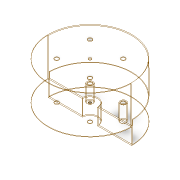
# Autodesk Inventor part: WaterproofCover
Saved by Autodesk Inventor 2018 (Build 220112000, 112)
## iProperties
Created: 2017-12-09
Part Number: WaterproofCover
Material: Polyethylene, Low Density
Document SubType Name: Modeling
Designer: Udara Wanasinghe
Mass: 493.701 g
Surface Area: 5556.42 cm^2
Volume: 552.239 cm^3
Density: 0.894 g/cm^3
Appearance: Smooth - Off-White
Author: Udara Wanasinghe
Autodesk Inventor part; units mm, degrees
ref_plane "YZ Plane" through (0, 0, 0) normal (1, 0, 0) x (0, 1, 0)
ref_plane "XZ Plane" through (0, 0, 0) normal (0, 1, 0) x (-1, 0, 0)
ref_plane "XY Plane" through (0, 0, 0) normal (0, 0, 1) x (1, 0, 0)
sketch "Sketch1" plane through (0, 0, 0) normal (0, 1, 0) x (-1, 0, 0)
  circle A0 centre (0, 0) radius 156
  dimension "d1" = 312
  constraints: 1 centre point
  measures "d1" diameter of A0
extrude "Extrusion1" add sketch "Sketch1" along normal blind 144
ref_plane "Work Plane1" through (0, 2, 0) normal (0, -1, 0) x (1, 0, 0)
sketch "Sketch2" plane through (0, 2, 0) normal (0, -1, 0) x (1, 0, 0)
  circle A0 centre (0, 0) radius 154
  dimension "d5" = 308
  constraints: 1 centre point, 1 coincident
  measures "d5" diameter of A0
extrude "Extrusion2" cut sketch "Sketch2" against normal blind 140
sketch "Sketch3" plane through (0, 144, 0) normal (0, 1, 0) x (1, 0, 0)
  circle A0 centre (0, 0) radius 5
  dimension "d8" = 10
  constraints: 1 centre point, 1 coincident
  measures "d8" diameter of A0
extrude "Extrusion3" cut sketch "Sketch3" against normal through all
sketch "Sketch5" plane through (0, 144, 0) normal (0, 1, 0) x (1, 0, 0)
  line L0 (0, 156) -> (0, -156) construction
  line L1 (156, 0) -> (-156, 0) construction
  circle A0 centre (62.132, -62.132) radius 7.5
  line L2 (62.132, -62.132) -> (0, -62.132) construction
  line L3 (62.132, -62.132) -> (62.132, 0) construction
  line L4 (62.132, -62.132) -> (106.066, -106.066) construction
  circle A1 centre (0, 0) radius 150 construction
  dimension "d20" = 300
  dimension "d17" = 312
  dimension "d18" = 312
  dimension "d19" = 15
  constraints: 10 end point, 2 coincident, 2 equal length, 2 midpoint, 2 perpendicular, 2 point on line, 1 centre point, 1 horizontal, 1 vertical, 4 other
  measures "d17" distance of L0.start L0.end
  measures "d18" distance of L1.start L1.end
  measures "d19" diameter of A0
extrude "Extrusion5" cut sketch "Sketch5" against normal through all
pattern_circular "Circular Pattern1" count 4 over 360 about axis through (0, -10, 0) along (0, 1, 0) of "Extrusion5"
sketch "Sketch4" plane through (0, 0, 0) normal (0, -1, 0) x (1, 0, 0)
  arc A0 (0, -156) -> (0, 156) centre (0, 0) ccw
  arc A1 (0, -28) -> (0, 28) centre (0, 0) ccw
  line L0 (0, -156) -> (0, -28)
  line L1 (0, 28) -> (0, 156)
  circle A2 centre (62.132, -62.132) radius 9.5
  circle A3 centre (62.132, -62.132) radius 7.5 projected
  circle A4 centre (62.132, 62.132) radius 9.5
  circle A5 centre (62.132, 62.132) radius 7.5 projected
  dimension "d11" = 312
  dimension "d12" = 56
  dimension "d26" = 19
  dimension "d27" = 19
  constraints: 4 centre point, 4 end point, 4 point on circle, 2 coincident, 2 concentric, 2 vertical
  measures "d11" diameter of A0
  measures "d12" diameter of A1
  measures "d26" diameter of A2
  measures "d27" diameter of A4
extrude "Extrusion6" add sketch "Sketch4" along normal blind 60 and the other way blind 2 contours L0 A1 L1 A0
ref_plane "Work Plane2" through (0, -58, 0) normal (0, -1, 0) x (1, 0, 0)
sketch "Sketch6" plane through (0, -58, 0) normal (0, -1, 0) x (1, 0, 0)
  arc A0 (3, -29.8496) -> (3, 29.8496) centre (0, 0) ccw
  circle A1 centre (62.132, 62.132) radius 11.5
  circle A2 centre (62.132, -62.132) radius 11.5
  circle A3 centre (62.132, 62.132) radius 7.5 projected
  circle A4 centre (62.132, -62.132) radius 7.5 projected
  line L0 (0, 149.3459) -> (0, -149.3522) construction
  line L1 (0, 28) -> (0, 156) construction
  arc A5 (3, -163.9369) -> (3, 163.9369) centre (0, 0) ccw
  arc A6 (0, -156) -> (0, 156) centre (0, 0) ccw projected
  line L2 (3, 163.9369) -> (3, 29.8496)
  line L3 (3, -29.8496) -> (3, -163.9369)
  arc A7 (0, -28) -> (0, 28) centre (0, 0) ccw projected
  dimension "d34" = 60
  dimension "d35" = 23
  dimension "d36" = 23
  constraints: 6 end point, 4 centre point, 4 concentric, 4 point on circle, 2 vertical, 1 collinear, 1 point on line
  measures "d34" diameter of A0
  measures "d35" diameter of A1
  measures "d36" diameter of A2
extrude "Extrusion7" cut sketch "Sketch6" against normal blind 80 contours A0 L2 A6 L3 | A6 L2 A5 L3
ref_plane "Work Plane3" through (0, 142, 0) normal (0, 1, 0) x (1, 0, 0)
sketch "Sketch7" plane through (0, 142, 0) normal (0, 1, 0) x (1, 0, 0)
  arc A0 (-2, 165.9507) -> (-2, -165.9507) centre (0, 0) ccw
  circle A1 centre (0, 0) radius 156 projected
  line L0 (-2, 165.9507) -> (-2, -165.9507)
  dimension "d41" = 2
  constraints: 2 end point, 2 point on circle, 1 centre point, 1 coincident, 1 concentric, 1 vertical
  measures "d41" distance from line of L0 point (0, 0)
extrude "Extrusion8" cut sketch "Sketch7" against normal blind 140 contours L0 A1 A0 | L0 A1 picked at (-54.0363, 21.9945)
body "Solid1"
